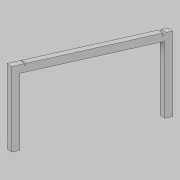
# Autodesk Inventor part: B0-ram
Saved by Autodesk Inventor 2018.1 (Build 221171000, 171)
## iProperties
Created: 2018-06-22
Part Number: B0-ram
Material: Všeobecné
Document SubType Name: Modeling
Designer: PS
Density: 1 g/cm^3
Appearance: Výchozí
Author: PS
Autodesk Inventor part; units mm, degrees
ref_plane "YZ Plane" through (0, 0, 0) normal (1, 0, 0) x (0, 1, 0)
ref_plane "XZ Plane" through (0, 0, 0) normal (0, 1, 0) x (-1, 0, 0)
ref_plane "XY Plane" through (0, 0, 0) normal (0, 0, 1) x (1, 0, 0)
sketch "Náčrt1" plane through (0, 0, 0) normal (0, 0, 1) x (1, 0, 0)
  line L0 (0, 0) -> (10000, 0)
  line L1 (10000, 0) -> (10000, 5000)
  line L2 (10000, 5000) -> (0, 5000)
  line L3 (0, 5000) -> (0, 0)
  line L4 (500, 0) -> (9500, 0)
  line L5 (9500, 0) -> (9500, 4500)
  line L6 (9500, 4500) -> (500, 4500)
  line L7 (500, 4500) -> (500, 0)
  dimension "d2" = 10000
  dimension "d3" = 500
  dimension "d4" = 500
  dimension "d5" = 500
  dimension "d6" = 5000
  constraints: 16 end point, 4 parallel, 2 horizontal, 2 perpendicular, 1 point on line
  measures "d2" distance of L1.end L2.end
  measures "d3" distance between parallel lines of L3 L7
  measures "d4" distance between parallel lines of L2 L6
  measures "d5" distance between parallel lines of L1 L5
  measures "d6" distance between parallel lines of L0 L2
extrude "Vysunutí1" add sketch "Náčrt1" along normal blind 500 contours L3 L2 L1 L0 L5 L6 L7
sketch "Náčrt3" plane through (0, 0, 500) normal (0, 0, 1) x (1, 0, 0)
  line L0 (10000, 5000) -> (0, 5000) projected
  line L1 (800, 5000) -> (900, 5000)
  line L2 (900, 5000) -> (800, 4900)
  line L3 (800, 4900) -> (800, 5000)
  line L4 (0, 5000) -> (0, 0) projected
  line L5 (9382.06, 5000) -> (9382.06, 4800)
  line L6 (9382.06, 4800) -> (9582.06, 5000)
  line L7 (9382.06, 5000) -> (9582.06, 5000)
  dimension "d15" = 100
  dimension "d16" = 800
  dimension "d19" = 45
  dimension "d20" = 8582.06
  dimension "d21" = 200
  constraints: 12 end point, 4 point on line, 2 perpendicular, 1 horizontal, 1 vertical
  measures "d15" distance of L2.end L1.start
  measures "d16" distance between parallel lines of L4 L3
  measures "d19" angle of L3 L2
  measures "d20" distance between parallel lines of L3 L5
  measures "d21" distance of L5.start L5.end
extrude "Vysunutí3" cut sketch "Náčrt3" against normal blind 587.25
equation "\"d4\" = d3"
equation "\"d5\" = d3"
